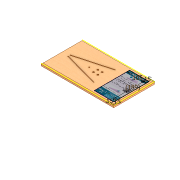
# Autodesk Inventor part: platform_instr
Saved by Autodesk Inventor 2020 (Build 240168000, 168)
## iProperties
Created: 2021-06-07
Part Number: platform_instr
Material: Generic
Document SubType Name: Modeling
Designer: Aidan Lee
Density: 1 g/cm^3
Appearance: Cherry - Natural Low Gloss
Author: Aidan Lee
Autodesk Inventor part; units mm, degrees
ref_plane "YZ Plane" through (0, 0, 0) normal (1, 0, 0) x (0, 1, 0)
ref_plane "XZ Plane" through (0, 0, 0) normal (0, 1, 0) x (-1, 0, 0)
ref_plane "XY Plane" through (0, 0, 0) normal (0, 0, 1) x (1, 0, 0)
sketch "Sketch1" plane through (0, 0, 0) normal (0, 1, 0) x (-1, 0, 0)
  line L0 (0, 0) -> (390, 0)
  line L1 (390, 0) -> (390, -219)
  line L2 (390, -219) -> (0, -219)
  line L3 (0, -219) -> (0, 0)
  dimension "d0" = 219
  dimension "d1" = 390
  constraints: 8 end point, 2 parallel, 1 horizontal, 1 perpendicular
  measures "d0" distance of L2.end L0.start
  measures "d1" distance of L0.start L0.end
extrude "Platform" add sketch "Sketch1" along normal blind 18
sketch "Sketch3" plane through (0, 18, 0) normal (0, 1, 0) x (1, 0, 0)
  circle A0 centre (-240.9586, 109.5) radius 3.1
  line L0 (0, 0) -> (0, 219) projected
  line L1 (-390, 0) -> (0, 0) projected
  line L2 (-229.5, 144) -> (-160.5, 144)
  line L3 (-160.5, 144) -> (-160.5, 75)
  line L4 (-160.5, 75) -> (-229.5, 75)
  line L5 (-229.5, 75) -> (-229.5, 144)
  line L6 (-206.5, 121) -> (-183.5, 98)
  circle A1 centre (-206.5, 121) radius 3.5
  circle A2 centre (-183.5, 98) radius 3.5
  circle A3 centre (-183.5, 121) radius 3.5
  circle A4 centre (-206.5, 98) radius 3.5
  line L7 (-206.5, 98) -> (-183.5, 121)
  point P0 (0, 109.5)
  point P1 (-195, 109.5)
  point P2 (-160.5, 109.5)
  point P3 (-195, 144)
  point P4 (0, 109.5)
  point P5 (-195, 0)
  dimension "screwdiameter" = 6.2
  dimension "d34" = 69
  dimension "d35" = 69
  dimension "d36" = 7
  dimension "d37" = 7
  dimension "d38" = 7
  dimension "d39" = 7
  dimension "d43" = 23
  constraints: 12 end point, 6 midpoint, 5 centre point, 5 horizontal alignment, 4 vertical alignment, 2 coincident, 2 parallel, 2 perpendicular, 1 horizontal
  measures "screwdiameter" diameter of A0
  measures "d34" distance of L2.start L2.end
  measures "d35" distance of L4.end L2.start
  measures "d36" diameter of A1
  measures "d37" diameter of A2
  measures "d38" diameter of A4
  measures "d39" diameter of A3
  measures "d43" distance from line of L2 L7.end
extrude "ScrewHole" cut sketch "Sketch3" against normal through all contours A0 | A3 | A2 | A4 | A1
sketch "Sketch2" plane through (0, 18, 0) normal (0, 1, 0) x (1, 0, 0)
  line L0 (-364.182, 109.5) -> (-365, 112.4901)
  line L1 (-365, 112.4901) -> (-145.0809, 172.6532)
  line L2 (-145.0809, 172.6532) -> (-144.2629, 169.6631)
  line L3 (-144.2629, 169.6631) -> (-364.182, 109.5)
  line L4 (0, 0) -> (0, 219) projected
  line L5 (18.6218, 109.5) -> (45.6135, 109.5)
  line L6 (-390, 0) -> (0, 0) projected
  line L7 (-364.182, 109.5) -> (-365, 106.5099)
  line L8 (-365, 106.5099) -> (-145.0809, 46.3468)
  line L9 (-145.0809, 46.3468) -> (-144.2629, 49.3369)
  line L10 (-144.2629, 49.3369) -> (-364.182, 109.5)
  line L11 (-350.5799, 116.435) -> (-349.7619, 113.4449)
  line L12 (-159.501, 168.7083) -> (-158.683, 165.7182)
  line L13 (-350.5799, 102.565) -> (-349.7619, 105.5551)
  line L14 (-159.501, 50.2917) -> (-158.683, 53.2818)
  line L15 (-390, 219) -> (-390, 0) projected
  point P0 (32.1177, 109.5)
  point P1 (0, 109.5)
  point P2 (-195, 0)
  point P3 (-254.2224, 139.5815)
  point P4 (-159.501, 50.2917)
  point P5 (-158.683, 53.2818)
  point P6 (-350.5799, 102.565)
  dimension "d6" = 3.1
  dimension "beta" = 15.3
  dimension "rail" = 228
  dimension "centre_offset" = 0
  dimension "offsetlength" = 14.95
  dimension "d20" = 14.95
  dimension "d44" = 198.1
  dimension "d52" = 25
  constraints: 26 end point, 8 symmetric about line, 5 perpendicular, 4 midpoint, 4 point on line, 1 horizontal, 1 horizontal alignment
  measures "d6" distance between parallel lines of L3 L1
  measures "beta" angle of L3 L5
  measures "rail" distance between parallel lines of L0 L2
  measures "centre_offset" distance from line of L0.start L5
  measures "offsetlength" distance between parallel lines of L0 L11
  measures "d20" distance between parallel lines of L2 L12
  measures "d44" distance between parallel lines of L12 L11
  measures "d52" distance from line of L15 L7.end
extrude "Slots" cut sketch "Sketch2" against normal blind 5 contours L11 L1 L12 L3 | L10 L14 L8 L13
chamfer "Chamfer1" distance 5 angle 45 8 edges at (-390, 18, -109.5) (-195, 18, 0) (-195, 18, -219) (0, 18, -109.5) (0, 0, -109.5) (-195, 0, 0) (-390, 0, -109.5) (-195, 0, -219)
chamfer "Countersunk" distance 1 angle 45 4 edges at (-210, 18, -98) (-210, 18, -121) (-187, 18, -121) (-187, 18, -98)
sketch "InstructionsSticker" plane through (0, 18, 0) normal (0, 1, 0) x (1, 0, 0)
  line L0 (-120, 15) -> (-15, 15)
  line L1 (-15, 15) -> (-15, 204)
  line L2 (-15, 204) -> (-120, 204)
  line L3 (-120, 204) -> (-120, 15)
  line L4 (0, 219) -> (-390, 219) projected
  line L5 (-390, 0) -> (0, 0) projected
  line L6 (0, 0) -> (0, 219) projected
  line L7 (-120, 204) -> (-15.0037, 204) construction
  line L8 (-15.0037, 204) -> (-15.0037, 14.9979) construction
  line L9 (-15.0037, 14.9979) -> (-120, 14.9979) construction
  line L10 (-120, 14.9979) -> (-120, 204) construction
  dimension "d53" = 105
  dimension "d54" = 15
  dimension "d55" = 15
  dimension "d56" = 15
  dimension "d58" = 189
  constraints: 8 end point, 2 parallel, 1 horizontal, 1 perpendicular, 2 other
  measures "d53" distance between parallel lines of L1 L3
  measures "d54" distance between parallel lines of L4 L2
  measures "d55" distance between parallel lines of L5 L0
  measures "d56" distance between parallel lines of L6 L1
  measures "d58" distance between parallel lines of L0 L2
equation "\"d20\" = offsetlength"
equation "\"gluegap\" = 0.1"
body "Solid1"
